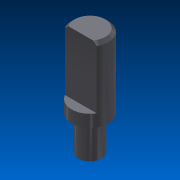
# Autodesk Inventor part: 12mm Incremental Encoder Shaft
Saved by Autodesk Inventor 2014 (Build 180170000, 170)
## iProperties
Created: 2011-11-08
Part Number: 12mm Incremental Encoder Shaft
Document SubType Name: Modeling
Designer: sdarley
Density: 1 g/cm^3
Material: Generic
Appearance: Steel - Polished
Author: sdarley
Autodesk Inventor part; units mm, degrees
ref_plane "YZ Plane" through (0, 0, 0) normal (1, 0, 0) x (0, 1, 0)
ref_plane "XZ Plane" through (0, 0, 0) normal (0, 1, 0) x (-1, 0, 0)
ref_plane "XY Plane" through (0, 0, 0) normal (0, 0, 1) x (1, 0, 0)
sketch "Sketch1" plane through (0, 0, 0) normal (0, 0, 1) x (1, 0, 0)
  circle A0 centre (0, 0) radius 2 projected
  circle A1 centre (0, 0) radius 3.5 projected
  circle A2 centre (0, 0) radius 1.9
  dimension "d0" = 3.8
  constraints: 1 centre point, 1 coincident
  measures "d0" diameter of A2
extrude "Extrusion1" add sketch "Sketch1" against normal blind 5 and the other way blind 0.5 contours A2
sketch "Sketch2" plane through (0, 0, 0.5) normal (0, 0, 1) x (1, 0, 0)
  circle A0 centre (0, 0) radius 1.9 projected
  circle A1 centre (0, 0) radius 3
  dimension "d3" = 6
  constraints: 1 centre point, 1 coincident
  measures "d3" diameter of A1
extrude "Extrusion2" add sketch "Sketch2" along normal blind 12 contours A0 | A1
sketch "Sketch3" plane through (0, 0, 12.5) normal (0, 0, 1) x (1, 0, 0)
  circle A0 centre (0, 0) radius 3 projected
  line L0 (-2.5981, -1.5) -> (2.5981, -1.5)
  dimension "d8" = 4.5
  constraints: 2 end point, 2 point on circle, 1 horizontal
extrude "Extrusion3" cut sketch "Sketch3" against normal blind 10 contours L0 A0 picked at (-0.7274, -1.6862)
chamfer "Chamfer1" distance 0.5 angle 45 2 edges at (2.8978, -0.7765, 12.5) (-0.7765, 2.8978, 12.5)
body "Solid1"
